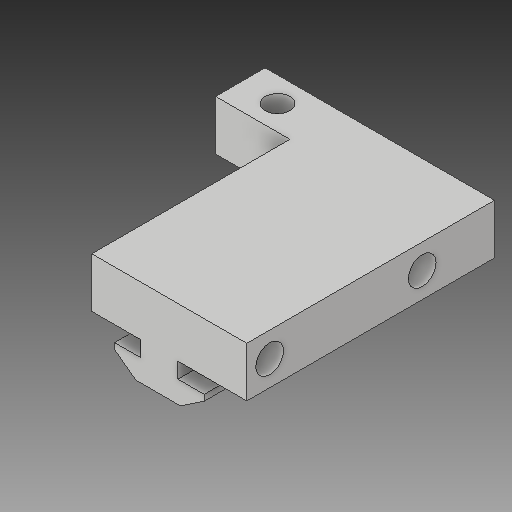
# Autodesk Inventor part: Sliderfor2020
Saved by Autodesk Inventor 2017 (Build 210142000, 142)
## iProperties
Created: 2017-12-08
Part Number: Sliderfor2020
Material: Generic
Document SubType Name: Modeling
Designer: User
Density: 1 g/cm^3
Appearance: Default
Mass: 5.11453 g
Surface Area: 33.3291 cm^2
Volume: 5.11453 cm^3
Author: User
Autodesk Inventor part; units mm, degrees
ref_plane "YZ Plane" through (0, 0, 0) normal (1, 0, 0) x (0, 1, 0)
ref_plane "XZ Plane" through (0, 0, 0) normal (0, 1, 0) x (-1, 0, 0)
ref_plane "XY Plane" through (0, 0, 0) normal (0, 0, 1) x (1, 0, 0)
sketch "Sketch1" plane through (0, 0, 0) normal (0, 0, 1) x (1, 0, 0)
  line L0 (0, 0) -> (14.5304, 0)
  line L1 (-8.7854, 6.6412) -> (11.0866, 6.6412)
  line L2 (11.0866, 1.6412) -> (2.2606, 1.6412)
  line L3 (2.2606, 1.6412) -> (2.2606, -0.3588)
  line L4 (2.2606, -0.3588) -> (5.6256, -0.3588)
  line L5 (2.5721, -3.1588) -> (-3.1429, -3.1588)
  line L6 (-3.1429, -3.1588) -> (-5.8644, -1.1208)
  line L7 (-5.8644, -1.1208) -> (-5.8644, -0.3588)
  line L8 (-5.8644, -0.3588) -> (-2.4994, -0.3588)
  line L9 (-2.4994, -0.3588) -> (-2.4994, 1.6412)
  line L10 (-2.4994, 1.6412) -> (-8.7854, 1.6412)
  line L11 (-8.7854, 1.6412) -> (-8.7854, 6.6412)
  line L12 (5.6256, -0.3588) -> (5.6256, -1.1208)
  line L13 (5.6256, -1.1208) -> (2.5721, -3.1588)
  line L14 (11.0866, 6.6412) -> (5.0156, 6.6412)
  line L15 (5.0156, 1.6412) -> (11.0866, 1.6412)
  line L16 (11.0866, 6.6412) -> (11.0866, 1.6412)
  dimension "d2" = 5
  dimension "d3" = 2
  dimension "d6" = 11.49
  dimension "d7" = 2.921
  dimension "d9" = 5.6425
  dimension "d11" = 0.762
  dimension "d12" = 0.762
  dimension "d78" = 5.461
  dimension "d88" = 3.365
  dimension "d89" = 3.365
  constraints: 34 end point, 5 perpendicular, 4 point on line, 3 horizontal, 2 vertical, 1 collinear
  measures "d2" distance between parallel lines of L10 L1
  measures "d3" distance between parallel lines of L8 L10
  measures "d6" distance between parallel lines of L7 L12
  measures "d7" distance between parallel lines of L7 L11
  measures "d9" distance from line of L5.end L11
  measures "d11" distance of L6.end L7.end
  measures "d12" distance of L4.end L12.end
  measures "d78" distance between parallel lines of L16 L12
  measures "d88" distance between parallel lines of L9 L7
  measures "d89" distance from line of L4.end L3
extrude "Extrusion1" add sketch "Sketch1" along normal blind 25.4
sketch "Sketch14" plane through (-8.7854, 1.6412, 0) normal (-1, 0, 0) x (0, 0, 1)
  line L0 (0, 0) -> (0, 5) projected
  line L1 (0, 0) -> (25.4, 0) projected
  line L2 (25.4, 5) -> (25.4, 0) projected
  line L3 (0, 5) -> (25.4, 5) projected
  line L4 (0, 5) -> (0, 0) projected
  line L5 (0, 0) -> (25.4, 0) projected
  line L6 (0, 5) -> (6.35, 5)
  line L7 (6.35, 5) -> (6.35, 0)
  line L8 (6.35, 0) -> (0, 0)
  line L9 (0, 0) -> (0, 5)
  point P0 (0, -1.6412)
  dimension "d161" = 6.35
  constraints: 8 end point, 2 parallel, 1 horizontal, 1 perpendicular, 1 point on line
  measures "d161" distance of L7.end L8.end
extrude "Extrusion6" add sketch "Sketch14" along normal blind 9.525 contours L0 L3 L7 L1
sketch "Sketch17" plane through (-8.7854, 6.6412, 25.4) normal (0, 1, 0) x (1, 0, 0)
  line L0 (-9.525, 25.4) -> (19.872, 25.4) projected
  line L1 (-9.525, 19.05) -> (-9.525, 25.4) projected
  line L2 (0, 19.05) -> (-9.525, 19.05) projected
  line L3 (0, 19.05) -> (0, 0) projected
  line L4 (19.872, 0) -> (0, 0) projected
  line L5 (19.872, 25.4) -> (19.872, 0) projected
  line L6 (-9.525, 25.4) -> (19.872, 25.4) projected
  line L7 (19.872, 0) -> (0, 0) projected
  line L8 (19.872, 25.4) -> (13.522, 25.4)
  line L9 (13.522, 0) -> (19.872, 0)
  line L10 (19.872, 0) -> (19.872, 25.4)
  point P0 (8.7854, 25.4)
  dimension "d175" = 6.35
  constraints: 6 end point, 1 horizontal, 1 parallel, 1 point on line
  measures "d175" distance of L9.end L9.start
extrude "Extrusion9" add sketch "Sketch17" along normal blind 1.397
sketch "Sketch19" plane through (-8.7854, 1.6412, 25.4) normal (0, -1, 0) x (1, 0, 0)
  line L0 (6.286, -25.4) -> (-9.525, -25.4) projected
  line L1 (6.286, -25.4) -> (6.286, 0) projected
  line L2 (0, 0) -> (6.286, 0) projected
  line L3 (0, -19.05) -> (0, 0) projected
  line L4 (0, -19.05) -> (-9.525, -19.05) projected
  line L5 (-9.525, -25.4) -> (-9.525, -19.05) projected
  point P0 (8.7854, -25.4)
  point P1 (-4.7625, -22.225)
hole "Hole11" at (-13.5479, 1.6412, 3.175) direction (0, 1, 0) diameter 3.175 depth 25.4 tip angle 118
sketch "Sketch20" plane through (0, 0, 25.4) normal (0, 0, 1) x (1, 0, 0)
  line L0 (-8.7854, 1.6412) -> (-8.7854, 8.0382) projected
  line L1 (-8.7854, 1.6412) -> (-2.4994, 1.6412) projected
  line L2 (-2.4994, 1.6412) -> (-2.4994, -0.3588) projected
  line L3 (-2.4994, -0.3588) -> (-5.8644, -0.3588) projected
  line L4 (-5.8644, -0.3588) -> (-5.8644, -1.1208) projected
  line L5 (-5.8644, -1.1208) -> (-3.1429, -3.1588) projected
  line L6 (-3.1429, -3.1588) -> (2.5721, -3.1588) projected
  line L7 (2.5721, -3.1588) -> (5.6256, -1.1208) projected
  line L8 (5.6256, -1.1208) -> (5.6256, -0.3588) projected
  line L9 (5.6256, -0.3588) -> (2.2606, -0.3588) projected
  line L10 (2.2606, -0.3588) -> (2.2606, 1.6412) projected
  line L11 (2.2606, 1.6412) -> (11.0866, 1.6412) projected
  line L12 (11.0866, 1.6412) -> (11.0866, 8.0382) projected
  line L13 (-8.7854, 8.0382) -> (11.0866, 8.0382) projected
  point P0 (0, 0)
extrude "Extrusion10" add sketch "Sketch20" along normal blind 6.35
sketch "Sketch21" plane through (11.0866, 1.6412, 0) normal (1, 0, 0) x (0, 0, -1)
  line L0 (0, 6.397) -> (0, 0) projected
  line L1 (0, 6.397) -> (-31.75, 6.397) projected
  line L2 (-31.75, 0) -> (-31.75, 6.397) projected
  line L3 (0, 0) -> (-31.75, 0) projected
  point P0 (0, -1.6412)
  point P1 (-28.829, 3.222)
  point P2 (-9.271, 3.222)
  dimension "d199" = 31.75
  dimension "d200" = 19.558
  dimension "d201" = 9.271
  dimension "d202" = 3.175
  dimension "d203" = 3.175
  measures "d199" distance of L0.start L1.end
  measures "d200" distance of point (-9.271, 3.222) point (-28.829, 3.222)
  measures "d201" distance from line of L0 point (-9.271, 3.222)
  measures "d202" distance from line of L1 point (-28.829, 3.222)
  measures "d203" distance from line of L1 point (-9.271, 3.222)
hole "Hole12" at (11.0866, 4.8632, 28.829) at (11.0866, 4.8632, 9.271) direction (-1, 0, 0) diameter 3.556 depth 25.4 tip angle 118
equation "\"d9\" = -0.5 * d8 + 0.5 * d0"
equation "\"d12\" = d11"
equation "\"d203\" = d202"
equation "\"d8\" = 5.715"
equation "\"d0\" = 17"
body "Solid1"
